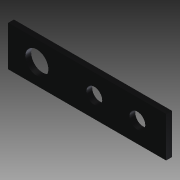
# Autodesk Inventor part: ZPT2_8_B_PLATE
Saved by Autodesk Inventor 2011 SP1 (Build 150282100, 282)
## iProperties
Created: 2018-01-08
Part Number: ZPT2_8_B_PLATE
Catalog Web Link: www.cadenas.de
Description: ZPT_2_8B_PLATE-Vacuum Pad/Vertical Vacuum Entry With Buffer
Vendor: SMC
Document SubType Name: Modeling
Designer: psAdmin
Manufacturer: SMC
Mass: 1.34444 g
Surface Area: 17.3982 cm^2
Volume: 1.34444 cm^3
Density: 1 g/cm^3
Category: PARTsolutions
Company: SMC
Title: ZPT2_8_B_PLATE
Author: Cadenas PARTsolutions
Comments: Vacuum Pad/Vertical Vacuum Entry With Buffer
PSOL_IDENT_0: {$CADENAS_DATA\23d-libs\smc_jp\vacuum_equipment\vacuum_pad\zp\zpt_b\zpt_2_8_b\parts\zpt_2_8_plate_b.
PSOL_IDENT_1: prj},178 {VTYP=3D},{NB=ZPT2_8_B_PLATE},{LINA=ZPT2_8_B_PLATE},{NN=ZPT_2_8B_PLATE},{DATE=12.07.2017 07
PSOL_IDENT_2: :16:19},{GEOMDATE=10.02.2011 00:00:00},{VERSION=},{LINEID=10},{LINESUBID=-1},{WBVAR=}  {NB=ZPT2_8_B_
PSOL_IDENT_3: PLATE},{LINA=ZPT2_8_B_PLATE},{KT=DUMMY},{ORDER=ZPT2_8}
NN: ZPT_2_8B_PLATE
NT: Vacuum Pad/Vertical Vacuum Entry With Buffer
NB: ZPT2_8_B_PLATE
NBSYN: $ORDER._B_PLATE
LINA: ZPT2_8_B_PLATE
ORDER: ZPT2_8
SUPPLIER: SMC
ARTICLENO: ZPT2_8_B_PLATE
BOMINFO: ZPT2_8_B_PLATE
CREATOR: CADENAS GmbH
Autodesk Inventor part; units mm, degrees
sketch "Sketch_1" plane through (0, 0, 0) normal (0, 1, 0) x (-1, 0, 0)
  line L0 (10, 7) -> (-45, 7)
  line L1 (-45, 7) -> (-45, -7)
  line L2 (-45, -7) -> (10, -7)
  line L3 (10, -7) -> (10, 7)
  circle A0 centre (-35, 0) radius 2.75
  circle A1 centre (-20, 0) radius 2.75
  circle A2 centre (0, 0) radius 4
  constraints: 8 end point, 3 centre point
extrude "Extrusion1" add sketch "Sketch_1" along normal mid plane 2
ref_plane "PLATE_BUFFER_XY" through (0, 0, 0) normal (0, -1, 0) x (1, 0, 0)
ref_plane "PLATE_BUFFER_YZ" through (0, 0, 0) normal (1, 0, 0) x (0, 0, 1)
ref_plane "PLATE_BUFFER_ZX" through (0, 0, 0) normal (0, 0, 1) x (0, -1, 0)
body "Solid1"
